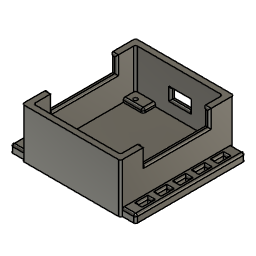
wristMount V1 (Autodesk Fusion 360 design; units mm, degrees)
Autodesk Fusion 360 part; units mm, degrees
sketch "Sketch1" plane through (0, 0, 0) normal (0, 0, 1) x (1, 0, 0)
  line L0 (26.02, 30.02) -> (-26.02, 30.02)
  line L1 (-26.02, 30.02) -> (-26.02, -30.02)
  line L2 (-26.02, -30.02) -> (26.02, -30.02)
  line L3 (26.02, -30.02) -> (26.02, 30.02)
  line L4 (26.02, 30.02) -> (-26.02, -30.02) construction
  line L5 (-26.02, 30.02) -> (26.02, -30.02) construction
  line L6 (-23.02, -27.02) -> (23.02, -27.02)
  line L7 (23.02, -27.02) -> (23.02, 27.02)
  line L8 (23.02, 27.02) -> (-23.02, 27.02)
  line L9 (-23.02, 27.02) -> (-23.02, -27.02)
  line L10 (19.25, 23.25) -> (-19.25, 23.25)
  line L11 (-19.25, 23.25) -> (-19.25, -23.25)
  line L12 (-19.25, -23.25) -> (19.25, -23.25)
  line L13 (19.25, -23.25) -> (19.25, 23.25)
  line L14 (19.25, 23.25) -> (-19.25, -23.25) construction
  line L15 (-19.25, 23.25) -> (19.25, -23.25) construction
  dimension "d1" = 52.04
  dimension "d2" = 60.04
  dimension "d3" = -3
  dimension "d4" = 46.5
  dimension "d5" = 38.5
  constraint horizontal L0
  constraint perpendicular L0 L1
  constraint parallel L0 L2
  constraint parallel L1 L3
  constraint coincident L4 origin
  constraint coincident L5 origin
  constraint horizontal L10
  constraint perpendicular L10 L11
  constraint parallel L10 L12
  constraint parallel L11 L13
  constraint coincident L14 origin
  constraint coincident L15 origin
  measures "d1" distance of L0.start L0.end
  measures "d2" distance of L0.end L1.end
  measures "d4" distance of L10.end L11.end
  measures "d5" distance of L10.start L10.end
extrude "Extrude1" add sketch "Sketch1" along normal blind 26.04 contours L0 L1 L2 L3 makes body 1
extrude "Extrude2" add sketch "Sketch1" along normal blind 3 contours L6 L7 L8 L9 | L10 L11 L12 L13 bodies 1
sketch "Sketch2" plane through (0, 0, 3) normal (0, 0, 1) x (-1, 0, 0)
  line L0 (23.02, -27.02) -> (23.02, 27.02)
  line L1 (23.02, 27.02) -> (-23.02, 27.02)
  line L2 (-23.02, 27.02) -> (-23.02, -27.02)
  line L3 (-23.02, -27.02) -> (23.02, -27.02)
  line L4 (23.02, -27.02) -> (12.52, -27.02)
  line L5 (12.52, -27.02) -> (12.52, -20.52)
  line L6 (12.52, -20.52) -> (23.02, -20.52)
  line L7 (23.02, -20.52) -> (23.02, -27.02)
  line L8 (-23.02, -27.02) -> (-12.52, -27.02)
  line L9 (-12.52, -27.02) -> (-12.52, -20.52)
  line L10 (-12.52, -20.52) -> (-23.02, -20.52)
  line L11 (-23.02, -20.52) -> (-23.02, -27.02)
  line L12 (23.02, 27.02) -> (12.52, 27.02)
  line L13 (12.52, 27.02) -> (12.52, 20.52)
  line L14 (12.52, 20.52) -> (23.02, 20.52)
  line L15 (23.02, 20.52) -> (23.02, 27.02)
  line L16 (-23.02, 27.02) -> (-12.52, 27.02)
  line L17 (-12.52, 27.02) -> (-12.52, 20.52)
  line L18 (-12.52, 20.52) -> (-23.02, 20.52)
  line L19 (-23.02, 20.52) -> (-23.02, 27.02)
  dimension "d10" = 10.5
  dimension "d11" = 6.5
  dimension "d12" = 6.5
  dimension "d13" = 10.5
  dimension "d14" = 6.5
  dimension "d15" = 10.5
  dimension "d16" = 10.5
  dimension "d17" = 6.5
  constraint horizontal L4
  constraint vertical L5
  constraint horizontal L6
  constraint vertical L7
  constraint coincident L0.start L3.end
  constraint horizontal L8
  constraint vertical L9
  constraint horizontal L10
  constraint vertical L11
  constraint coincident L2.end L3.start
  constraint horizontal L12
  constraint vertical L13
  constraint horizontal L14
  constraint vertical L15
  constraint coincident L0.end L1.start
  constraint horizontal L16
  constraint vertical L17
  constraint horizontal L18
  constraint vertical L19
  constraint coincident L1.end L2.start
  measures "d10" distance of L5.end L6.end
  measures "d11" distance of L4.end L5.end
  measures "d12" distance of L8.end L9.end
  measures "d13" distance of L9.end L10.end
  measures "d14" distance of L12.end L13.end
  measures "d15" distance of L13.end L14.end
  measures "d16" distance of L17.end L18.end
  measures "d17" distance of L16.end L17.end
extrude "Extrude3" add sketch "Sketch2" along normal blind 2 contours L0 L3 L4 L5 L6 L7 bodies 1
extrude "Extrude4" add sketch "Sketch2" along normal blind 2 contours L2 L3 L8 L9 L10 L11 bodies 1
extrude "Extrude5" add sketch "Sketch2" along normal blind 2 contours L1 L2 L16 L17 L18 L19 bodies 1
extrude "Extrude6" add sketch "Sketch2" along normal blind 2 contours L0 L1 L12 L13 L14 L15 bodies 1
fillet "Fillet1" radius 1 1 edges at (12.52, -23.77, 5) on bodies 1
fillet "Fillet2" radius 1 1 edges at (-12.52, -23.77, 5) on bodies 1
fillet "Fillet3" radius 1 3 edges at (18.27, -20.52, 5) (12.8129, -20.52, 4.7071) (12.52, -20.52, 3.5) on bodies 1
fillet "Fillet4" radius 1 3 edges at (-12.52, -20.52, 3.5) (-12.8129, -20.52, 4.7071) (-18.27, -20.52, 5) on bodies 1
fillet "Fillet5" radius 1 1 edges at (-17.77, 20.52, 5) on bodies 1
fillet "Fillet6" radius 1 3 edges at (-12.52, 20.52, 3.5) (-12.52, 20.8129, 4.7071) (-12.52, 24.27, 5) on bodies 1
fillet "Fillet7" radius 1 1 edges at (12.52, 23.77, 5) on bodies 1
fillet "Fillet8" radius 1 3 edges at (12.52, 20.52, 3.5) (12.8129, 20.52, 4.7071) (18.27, 20.52, 5) on bodies 1
fillet "Fillet9" radius 1 2 edges at (-23.02, 27.02, 15.52) (-26.02, -30.02, 13.02) on bodies 1
fillet "Fillet10" radius 1 1 edges at (26.02, -30.02, 13.02) on bodies 1
fillet "Fillet11" radius 1 1 edges at (26.02, 30.02, 13.02) on bodies 1
fillet "Fillet12" radius 1 1 edges at (-26.02, 30.02, 13.02) on bodies 1
hole "Hole1" at (19.25, 23.25, 0) at (-19.25, 23.25, 0) at (-19.25, -23.25, 0) at (19.25, -23.25, 0) direction (0, 0, 1) diameter 2.04 depth 15 tip angle 118 bodies 1
fillet "Fillet13" radius 1 1 edges at (23.02, -27.02, 15.52) on bodies 1
fillet "Fillet14" radius 1 1 edges at (-23.02, -27.02, 15.52) on bodies 1
fillet "Fillet15" radius 1 1 edges at (23.02, 27.02, 15.52) on bodies 1
sketch "Sketch5" plane through (0, 0, 26.04) normal (0, 0, 1) x (-1, 0, 0)
  arc A0 (25.02, -30.02) -> (26.02, -29.02) centre (25.02, -29.02) ccw
  line L0 (26.02, -29.02) -> (26.02, 29.02)
  arc A1 (26.02, 29.02) -> (25.02, 30.02) centre (25.02, 29.02) ccw
  line L1 (25.02, 30.02) -> (-25.02, 30.02)
  arc A2 (-25.02, 30.02) -> (-26.02, 29.02) centre (-25.02, 29.02) ccw
  line L2 (-26.02, 29.02) -> (-26.02, -29.02)
  arc A3 (-26.02, -29.02) -> (-25.02, -30.02) centre (-25.02, -29.02) ccw
  line L3 (-25.02, -30.02) -> (25.02, -30.02)
  line L4 (23.02, 26.02) -> (23.02, -26.02)
  arc A4 (22.02, -27.02) -> (23.02, -26.02) centre (22.02, -26.02) ccw
  line L5 (22.02, -27.02) -> (-22.02, -27.02)
  arc A5 (-23.02, -26.02) -> (-22.02, -27.02) centre (-22.02, -26.02) ccw
  line L6 (-23.02, -26.02) -> (-23.02, 26.02)
  arc A6 (-22.02, 27.02) -> (-23.02, 26.02) centre (-22.02, 26.02) ccw
  line L7 (-22.02, 27.02) -> (22.02, 27.02)
  arc A7 (23.02, 26.02) -> (22.02, 27.02) centre (22.02, 26.02) ccw
  line L8 (26.02, 17) -> (-26.02, 17)
  line L9 (-26.02, 17) -> (-26.02, -17)
  line L10 (-26.02, -17) -> (26.02, -17)
  line L11 (26.02, -17) -> (26.02, 17)
  line L12 (26.02, 17) -> (-26.02, -17) construction
  line L13 (-26.02, 17) -> (26.02, -17) construction
  dimension "d59" = 10.02
  constraint horizontal L8
  constraint perpendicular L8 L9
  constraint parallel L8 L10
  constraint parallel L9 L11
  constraint coincident L12 origin
  constraint coincident L13 origin
  constraint coincident L0 L8.start
  measures "d59" distance of L7 L8
extrude "Extrude7" cut sketch "Sketch5" against normal blind 8.6 contours L0 L4 L8 L10 L11 | L2 L6 L8 L9 L10 bodies 1
fillet "Fillet16" radius 1 16 edges at (26.02, -17, 21.74) (24.52, -17, 26.04) (23.02, -17, 21.74) (26.02, 0, 17.44) (23.02, 0, 17.44) (-23.02, -17, 21.74) (-26.02, -17, 21.74) (-24.52, -17, 26.04) (-23.02, 0, 17.44) (-26.02, 0, 17.44) (26.02, 17, 21.74) (-23.02, 17, 21.74) (23.02, 17, 21.74) (-26.02, 17, 21.74) (24.52, 17, 26.04) (-24.52, 17, 26.04) on bodies 1
sketch "Sketch7" plane through (0, 27.02, 0) normal (0, -1, 0) x (1, 0, 0)
  line L0 (22.02, 5) -> (22.02, 26.04)
  line L1 (22.02, 26.04) -> (-22.02, 26.04)
  line L2 (-22.02, 26.04) -> (-22.02, 5)
  line L3 (-22.02, 5) -> (-13.52, 5)
  arc A0 (-12.52, 4) -> (-13.52, 5) centre (-13.52, 4) ccw
  line L4 (-12.52, 4) -> (-12.52, 3)
  line L5 (-12.52, 3) -> (12.52, 3)
  line L6 (12.52, 3) -> (12.52, 4)
  arc A1 (13.52, 5) -> (12.52, 4) centre (13.52, 4) ccw
  line L7 (13.52, 5) -> (22.02, 5)
  line L8 (5.5, 15) -> (-4.5, 15)
  line L9 (-4.5, 15) -> (-4.5, 10)
  line L10 (-4.5, 10) -> (5.5, 10)
  line L11 (5.5, 10) -> (5.5, 15)
  line L12 (5.5, 15) -> (-4.5, 10) construction
  line L13 (-4.5, 15) -> (5.5, 10) construction
  point P0 (0.5, 12.5)
  dimension "d64" = 10
  dimension "d65" = 16.52
  dimension "d66" = 7
  dimension "d71" = 5
  constraint horizontal L8
  constraint perpendicular L8 L9
  constraint parallel L8 L10
  constraint parallel L9 L11
  constraint coincident L12 P0
  constraint coincident L13 P0
  measures "d64" distance of L8.start L8.end
  measures "d65" distance of L0 L11
  measures "d66" distance of L5 L10
  measures "d71" distance of L8.end L9.end
extrude "Extrude8" cut sketch "Sketch7" against normal blind 3 contours L8 L9 L10 L11 bodies 1
fillet "Fillet17" radius 1 8 edges at (0.5, 27.02, 10) (0.5, 30.02, 10) (0.5, 27.02, 15) (-4.5, 27.02, 12.5) (5.5, 27.02, 12.5) (0.5, 30.02, 15) (5.5, 30.02, 12.5) (-4.5, 30.02, 12.5) on bodies 1
sketch "Sketch9" plane through (0, 0, 26.04) normal (0, 0, 1) x (-1, 0, 0)
  line L0 (23.02, -18) -> (23.02, -26.02)
  arc A0 (22.02, -27.02) -> (23.02, -26.02) centre (22.02, -26.02) ccw
  line L1 (22.02, -27.02) -> (-22.02, -27.02)
  arc A1 (-23.02, -26.02) -> (-22.02, -27.02) centre (-22.02, -26.02) ccw
  line L2 (-23.02, -26.02) -> (-23.02, -18)
  line L3 (-26.02, -18) -> (-26.02, -29.02)
  arc A2 (-26.02, -29.02) -> (-25.02, -30.02) centre (-25.02, -29.02) ccw
  line L4 (-25.02, -30.02) -> (25.02, -30.02)
  arc A3 (25.02, -30.02) -> (26.02, -29.02) centre (25.02, -29.02) ccw
  line L5 (26.02, -29.02) -> (26.02, -18)
  line L6 (26.02, -30.02) -> (-26.02, -30.02)
  line L7 (-26.02, -30.02) -> (-26.02, 30.02)
  line L8 (-26.02, 30.02) -> (26.02, 30.02)
  line L9 (26.02, 30.02) -> (26.02, -30.02)
  line L10 (26.02, -18) -> (23.02, -18)
  line L11 (-23.02, -18) -> (-26.02, -18)
  dimension "d74" = 52.04
  dimension "d75" = 60.04
  constraint horizontal L6
  constraint vertical L7
  constraint horizontal L8
  constraint vertical L9
  measures "d74" distance of L6.start L6.end
  measures "d75" distance of L6.start L8.end
sketch "Sketch10" plane through (0, 0, 26.04) normal (0, 0, 1) x (-1, 0, 0)
  line L0 (26.02, -18) -> (23.02, -18)
  line L1 (23.02, -18) -> (23.02, -26.02)
  arc A0 (22.02, -27.02) -> (23.02, -26.02) centre (22.02, -26.02) ccw
  line L2 (22.02, -27.02) -> (-22.02, -27.02)
  arc A1 (-23.02, -26.02) -> (-22.02, -27.02) centre (-22.02, -26.02) ccw
  line L3 (-23.02, -26.02) -> (-23.02, -18)
  line L4 (-23.02, -18) -> (-26.02, -18)
  line L5 (-26.02, -18) -> (-26.02, -29.02)
  arc A2 (-26.02, -29.02) -> (-25.02, -30.02) centre (-25.02, -29.02) ccw
  line L6 (-25.02, -30.02) -> (25.02, -30.02)
  arc A3 (25.02, -30.02) -> (26.02, -29.02) centre (25.02, -29.02) ccw
  line L7 (26.02, -29.02) -> (26.02, -18)
  line L8 (-26.02, -30.02) -> (26.02, -30.02)
  line L9 (26.02, -30.02) -> (26.02, 30.02)
  line L10 (26.02, 30.02) -> (-26.02, 30.02)
  line L11 (-26.02, 30.02) -> (-26.02, -30.02)
  line L12 (-26.02, -30.02) -> (26.02, 30.02) construction
  line L13 (26.02, -30.02) -> (-26.02, 30.02) construction
  line L14 (21.98, 27) -> (-22.02, 27)
  line L15 (-23.02, 26) -> (-23.02, -26)
  line L16 (-22.02, -27) -> (21.98, -27)
  line L17 (22.98, -26) -> (22.98, 26)
  arc A4 (21.98, -27) -> (22.98, -26) centre (21.98, -26) ccw
  arc A5 (-23.02, -26) -> (-22.02, -27) centre (-22.02, -26) ccw
  arc A6 (-22.02, 27) -> (-23.02, 26) centre (-22.02, 26) ccw
  arc A7 (22.98, 26) -> (21.98, 27) centre (21.98, 26) ccw
  line L18 (-19.25, -23.25) -> (19.25, -23.25)
  line L19 (19.25, -23.25) -> (19.25, 23.25)
  line L20 (19.25, 23.25) -> (-19.25, 23.25)
  line L21 (-19.25, 23.25) -> (-19.25, -23.25)
  line L22 (-19.25, -23.25) -> (19.25, 23.25) construction
  line L23 (19.25, -23.25) -> (-19.25, 23.25) construction
  point P0 (-23.02, 27)
  point P1 (-23.02, -27)
  point P2 (22.98, -27)
  dimension "d78" = 54
  dimension "d79" = 46
  dimension "d80" = 1
  dimension "d89" = 46.5
  dimension "d90" = 38.5
  constraint horizontal L8
  constraint perpendicular L8 L9
  constraint parallel L8 L10
  constraint parallel L9 L11
  constraint coincident L12 origin
  constraint coincident L13 origin
  constraint horizontal L14
  constraint vertical L15
  constraint horizontal L16
  constraint vertical L17
  constraint coincident P2 L16
  constraint coincident P2 L17
  constraint tangent L16 A4
  constraint tangent L17 A4
  constraint coincident P1 L15
  constraint coincident P1 L16
  constraint tangent L15 A5
  constraint tangent L16 A5
  constraint equal A4 A5
  constraint coincident P0 L14
  constraint coincident P0 L15
  constraint tangent L14 A6
  constraint tangent L15 A6
  constraint equal A4 A6
  constraint tangent L14 A7
  constraint tangent L17 A7
  constraint equal A4 A7
  constraint horizontal L18
  constraint perpendicular L18 L19
  constraint parallel L18 L20
  constraint parallel L19 L21
  constraint coincident L22 origin
  constraint coincident L23 origin
  measures "d78" distance of P0 P1
  measures "d79" distance of P1 P2
  measures "d80" radius of A4
  measures "d89" distance of L18.end L19.end
  measures "d90" distance of L18.start L18.end
extrude "Extrude10" add sketch "Sketch10" along normal blind 3 separate body contours L0 L1 A0 L2 A1 L3 L4 L5 A2 L6 A3 L7 L8 L9 L11 L15 A5 | L0 L1 A0 L2 A1 L4 L9 L10 L11 L14 L15 L16 L17 A4 A5 A6 A7 | L3 L14 L15 L16 L17 A4 A5 A6 A7 | L18 L19 L20 L21 makes body 2
extrude "Extrude11" add sketch "Sketch10" against normal blind 3 contours L3 L14 L15 L16 L17 A4 A5 A6 A7 | L18 L19 L20 L21 bodies 2
fillet "Fillet18" radius 1 1 edges at (-26.02, -30.02, 27.54) on bodies 2
fillet "Fillet19" radius 1 1 edges at (26.02, -30.02, 27.54) on bodies 2
hole "Hole2" at (-19.25, 23.25, 26.04) at (19.25, 23.25, 26.04) at (19.25, -23.25, 26.04) at (-19.25, -23.25, 26.04) direction (0, 0, 1) diameter 5 depth 3 tip angle 118 bodies 2
hole "Hole3" at (-19.25, 23.25, 26.04) at (19.25, -23.25, 26.04) at (-19.25, -23.25, 26.04) at (19.25, 23.25, 26.04) direction (0, 0, -1) diameter 2.04 depth 3 tip angle 118 bodies 2
hole "Hole4" at (-19.25, -23.25, 0) at (19.25, -23.25, 0) at (19.25, 23.25, 0) at (-19.25, 23.25, 0) direction (0, 0, 1) diameter 5 depth 1 tip angle 180 bodies 1
sketch "Sketch11" plane through (26.02, 0, 0) normal (1, 0, 0) x (0, 1, 0)
  line L0 (18, 26.04) -> (18, 16.44)
  line L1 (18, 16.44) -> (-18, 16.44)
  line L2 (-18, 16.44) -> (-18, 26.04)
  line L3 (-18, 26.04) -> (-29.02, 26.04)
  line L4 (-29.02, 26.04) -> (-29.02, 0)
  line L5 (-29.02, 0) -> (29.02, 0)
  line L6 (29.02, 0) -> (29.02, 26.04)
  line L7 (29.02, 26.04) -> (18, 26.04)
  line L8 (-29.02, 0) -> (29, 0)
  line L9 (29, 0) -> (29, 4)
  line L10 (29, 4) -> (-29.02, 4)
  line L11 (-29.02, 4) -> (-29.02, 0)
  constraint horizontal L8
  constraint vertical L9
  constraint horizontal L10
  constraint vertical L11
  constraint coincident L4.end L5.start
extrude "Extrude12" add sketch "Sketch11" along normal blind 7 contours L4 L5 L8 L9 L10 L11 bodies 1
sketch "Sketch12" plane through (-26.02, 0, 0) normal (-1, 0, 0) x (0, -1, 0)
  line L0 (-18, 16.44) -> (-18, 26.04)
  line L1 (-18, 26.04) -> (-29.02, 26.04)
  line L2 (-29.02, 26.04) -> (-29.02, 0)
  line L3 (-29.02, 0) -> (29.02, 0)
  line L4 (29.02, 0) -> (29.02, 26.04)
  line L5 (29.02, 26.04) -> (18, 26.04)
  line L6 (18, 26.04) -> (18, 16.44)
  line L7 (18, 16.44) -> (-18, 16.44)
  line L8 (-29.02, 0) -> (29.02, 0)
  line L9 (29.02, 0) -> (29.02, 4)
  line L10 (29.02, 4) -> (-29.02, 4)
  line L11 (-29.02, 4) -> (-29.02, 0)
  dimension "d102" = 4
  constraint horizontal L8
  constraint vertical L9
  constraint horizontal L10
  constraint vertical L11
  constraint coincident L4 L9.end
  constraint coincident L2.end L3.start
  measures "d102" distance of L2.end L10.end
extrude "Extrude13" add sketch "Sketch12" along normal blind 7 contours L2 L3 L4 L8 L9 L10 L11 bodies 1
sketch "Sketch13" plane through (0, 0, 4) normal (0, 0, 1) x (-1, 0, 0)
  line L0 (-26.02, -29) -> (-26.02, 29.02)
  line L1 (-26.02, 29.02) -> (-33.02, 29.02)
  line L2 (-33.02, 29.02) -> (-33.02, -29)
  line L3 (-33.02, -29) -> (-26.02, -29)
  line L4 (30, -22.5) -> (28, -22.5)
  line L5 (28, -22.5) -> (28, -17.5)
  line L6 (28, -17.5) -> (30, -17.5)
  line L7 (30, -17.5) -> (30, -22.5)
  line L8 (30, -12.5) -> (28, -12.5)
  line L9 (28, -12.5) -> (28, -7.5)
  line L10 (28, -7.5) -> (30, -7.5)
  line L11 (30, -7.5) -> (30, -12.5)
  line L12 (30, -2.5) -> (28, -2.5)
  line L13 (28, -2.5) -> (28, 2.5)
  line L14 (28, 2.5) -> (30, 2.5)
  line L15 (30, 2.5) -> (30, -2.5)
  line L16 (30, 7.5) -> (28, 7.5)
  line L17 (28, 7.5) -> (28, 12.5)
  line L18 (28, 12.5) -> (30, 12.5)
  line L19 (30, 12.5) -> (30, 7.5)
  line L20 (30, 17.5) -> (28, 17.5)
  line L21 (28, 17.5) -> (28, 22.5)
  line L22 (28, 22.5) -> (30, 22.5)
  line L23 (30, 22.5) -> (30, 17.5)
  line L24 (-28, -22.5) -> (-30, -22.5)
  line L25 (-30, -22.5) -> (-30, -17.5)
  line L26 (-30, -17.5) -> (-28, -17.5)
  line L27 (-28, -17.5) -> (-28, -22.5)
  line L28 (-28, -12.5) -> (-30, -12.5)
  line L29 (-30, -12.5) -> (-30, -7.5)
  line L30 (-30, -7.5) -> (-28, -7.5)
  line L31 (-28, -7.5) -> (-28, -12.5)
  line L32 (-28, -2.5) -> (-30, -2.5)
  line L33 (-30, -2.5) -> (-30, 2.5)
  line L34 (-30, 2.5) -> (-28, 2.5)
  line L35 (-28, 2.5) -> (-28, -2.5)
  line L36 (-28, 7.5) -> (-30, 7.5)
  line L37 (-30, 7.5) -> (-30, 12.5)
  line L38 (-30, 12.5) -> (-28, 12.5)
  line L39 (-28, 12.5) -> (-28, 7.5)
  line L40 (-28, 17.5) -> (-30, 17.5)
  line L41 (-30, 17.5) -> (-30, 22.5)
  line L42 (-30, 22.5) -> (-28, 22.5)
  line L43 (-28, 22.5) -> (-28, 17.5)
  dimension "d105" = 2
  dimension "d106" = 5
  dimension "d107" = 5
  dimension "d108" = 2
  dimension "d109" = 2
  dimension "d110" = 5
  dimension "d111" = 5
  dimension "d112" = 2
  dimension "d113" = 5
  dimension "d114" = 2
  dimension "d115" = 2
  dimension "d116" = 5
  dimension "d117" = 2
  dimension "d118" = 5
  dimension "d119" = 5
  dimension "d120" = 2
  dimension "d121" = 2
  dimension "d122" = 5
  dimension "d123" = 2
  dimension "d124" = 5
  dimension "d125" = 0
  constraint horizontal L4
  constraint vertical L5
  constraint horizontal L6
  constraint vertical L7
  constraint horizontal L8
  constraint vertical L9
  constraint horizontal L10
  constraint vertical L11
  constraint horizontal L12
  constraint vertical L13
  constraint horizontal L14
  constraint vertical L15
  constraint horizontal L16
  constraint vertical L17
  constraint horizontal L18
  constraint vertical L19
  constraint horizontal L20
  constraint vertical L21
  constraint horizontal L22
  constraint vertical L23
  constraint horizontal L24
  constraint vertical L25
  constraint horizontal L26
  constraint vertical L27
  constraint horizontal L28
  constraint vertical L29
  constraint horizontal L30
  constraint vertical L31
  constraint horizontal L32
  constraint vertical L33
  constraint horizontal L34
  constraint vertical L35
  constraint horizontal L36
  constraint vertical L37
  constraint horizontal L38
  constraint vertical L39
  constraint horizontal L40
  constraint vertical L41
  constraint horizontal L42
  constraint vertical L43
  measures "d105" distance of L4.start L4.end
  measures "d106" distance of L4.start L6.end
  measures "d107" distance of L8.start L10.end
  measures "d108" distance of L8.start L8.end
  measures "d109" distance of L12.start L12.end
  measures "d110" distance of L12.start L14.end
  measures "d111" distance of L16.start L18.end
  measures "d112" distance of L16.start L16.end
  measures "d113" distance of L20.start L22.end
  measures "d114" distance of L20.start L20.end
  measures "d115" distance of L24.start L24.end
  measures "d116" distance of L24.start L26.end
  measures "d117" distance of L28.start L28.end
  measures "d118" distance of L28.start L30.end
  measures "d119" distance of L32.start L34.end
  measures "d120" distance of L32.start L32.end
  measures "d121" distance of L36.start L36.end
  measures "d122" distance of L36.start L38.end
  measures "d123" distance of L40.start L40.end
  measures "d124" distance of L40.start L42.end
  measures "d125" distance of L19 L23
extrude "Extrude14" cut sketch "Sketch13" against normal blind 5 contours L4 L5 L6 L7 | L8 L9 L10 L11 | L12 L13 L14 L15 | L16 L17 L18 L19 | L20 L21 L22 L23 | L24 L25 L26 L27 | L28 L29 L30 L31 | L32 L33 L34 L35 | L36 L37 L38 L39 | L40 L41 L42 L43 bodies 1
fillet "Fillet20" radius 1 25 edges at (-33.02, 29.02, 2) (-29.52, 29.02, 4) (-30, 10, 4) (-28, 10, 4) (-29, 12.5, 4) (-29, 17.5, 4) (-30, 20, 4) (-29, 22.5, 4) (-28, 20, 4) (-28, -10, 4) (-29, -7.5, 4) (-30, -10, 4) (-29, -12.5, 4) (-30, -20, 4) (-29, -22.5, 4) (-28, -20, 4) (-29, -17.5, 4) (-28, 0, 4) (-29, 2.5, 4) (-30, 0, 4) (-29, -2.5, 4) (-29, 7.5, 4) (-33.02, 0, 4) (-29.52, -29.02, 4) (-33.02, -29.02, 2) on bodies 1
fillet "Fillet21" radius 1 20 edges at (-28, -20, 0) (-29, -22.5, 0) (-30, -20, 0) (-29, -17.5, 0) (-29, -12.5, 0) (-28, -10, 0) (-29, -7.5, 0) (-30, -10, 0) (-29, -2.5, 0) (-28, 0, 0) (-29, 2.5, 0) (-30, 0, 0) (-29, 7.5, 0) (-28, 10, 0) (-29, 12.5, 0) (-30, 10, 0) (-29, 17.5, 0) (-28, 20, 0) (-29, 22.5, 0) (-30, 20, 0) on bodies 1
fillet "Fillet22" radius 1 25 edges at (30, -20, 4) (29, -22.5, 4) (28, -20, 4) (29, -17.5, 4) (29, -12.5, 4) (28, -10, 4) (29, -7.5, 4) (30, -10, 4) (28, 0, 4) (29, -2.5, 4) (30, 0, 4) (29, 2.5, 4) (28, 10, 4) (29, 7.5, 4) (30, 10, 4) (29, 12.5, 4) (28, 20, 4) (29, 17.5, 4) (30, 20, 4) (29, 22.5, 4) (29.52, -29.02, 4) (33.02, -29.02, 2) (33.02, -0.01, 4) (33.02, 29, 2) (29.52, 29, 4) on bodies 1
fillet "Fillet23" radius 1 20 edges at (29, 22.5, 0) (30, 20, 0) (28, 20, 0) (29, 17.5, 0) (30, 10, 0) (29, 12.5, 0) (28, 10, 0) (29, 7.5, 0) (30, 0, 0) (29, 2.5, 0) (28, 0, 0) (29, -2.5, 0) (30, -10, 0) (29, -7.5, 0) (28, -10, 0) (29, -12.5, 0) (30, -20, 0) (29, -17.5, 0) (28, -20, 0) (29, -22.5, 0) on bodies 1
sketch "Sketch14" plane through (0, 0, 23.04) normal (0, 0, -1) x (1, 0, 0)
  circle A0 centre (-19.25, 23.25) radius 1.02
  circle A1 centre (-19.25, -23.25) radius 1.02
  circle A2 centre (19.25, 23.25) radius 1.02
  circle A3 centre (19.25, -23.25) radius 1.02
  arc A4 (-21.98, 27) -> (-22.98, 26) centre (-21.98, 26) ccw
  line L0 (-22.98, 26) -> (-22.98, -26)
  arc A5 (-22.98, -26) -> (-21.98, -27) centre (-21.98, -26) ccw
  line L1 (-21.98, -27) -> (22.02, -27)
  arc A6 (22.02, -27) -> (23.02, -26) centre (22.02, -26) ccw
  line L2 (23.02, -26) -> (23.02, 26)
  arc A7 (23.02, 26) -> (22.02, 27) centre (22.02, 26) ccw
  line L3 (22.02, 27) -> (-21.98, 27)
  line L4 (23.02, 20.5) -> (-23.02, 20.5)
  line L5 (-23.02, 20.5) -> (-23.02, -20.5)
  line L6 (-23.02, -20.5) -> (23.02, -20.5)
  line L7 (23.02, -20.5) -> (23.02, 20.5)
  line L8 (23.02, 20.5) -> (-23.02, -20.5) construction
  line L9 (-23.02, 20.5) -> (23.02, -20.5) construction
  line L10 (8.02, 27) -> (-8.02, 27)
  line L11 (-8.02, 27) -> (-8.02, -27)
  line L12 (-8.02, -27) -> (8.02, -27)
  line L13 (8.02, -27) -> (8.02, 27)
  line L14 (8.02, 27) -> (-8.02, -27) construction
  line L15 (-8.02, 27) -> (8.02, -27) construction
  dimension "d136" = 6.5
  dimension "d137" = 15
  constraint horizontal L4
  constraint perpendicular L4 L5
  constraint parallel L4 L6
  constraint parallel L5 L7
  constraint coincident L8 origin
  constraint coincident L9 origin
  constraint coincident L2 L4.start
  constraint horizontal L10
  constraint perpendicular L10 L11
  constraint parallel L10 L12
  constraint parallel L11 L13
  constraint coincident L14 origin
  constraint coincident L15 origin
  constraint coincident L3 L10.start
  measures "d136" distance of L3 L4
  measures "d137" distance of L7 L13
extrude "Extrude15" cut sketch "Sketch14" against normal blind 3 contours L3 L4 L10 L11 L13 | L0 L4 L6 L11 | L4 L6 L11 L13 | L2 L4 L6 L7 L13 | L1 L6 L11 L12 L13 bodies 2
fillet "Fillet24" radius 1 11 edges at (-22.98, 20.5, 24.54) (-8.02, 27, 24.54) (8.02, 27, 24.54) (8.02, 20.5, 24.54) (8.02, -20.5, 24.54) (8.02, -27, 24.54) (23.02, -20.5, 24.54) (-8.02, -20.5, 24.54) (-22.98, -20.5, 24.54) (-8.02, -27, 24.54) (-8.02, 20.5, 24.54) on bodies 2
fillet "Fillet25" radius 1 1 edges at (23.02, 20.5, 24.54) on bodies 2
hidden bodies 2
named bodies: "Box", "Lid"
